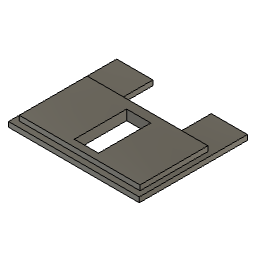
table_window (Autodesk Fusion 360 design; units mm, degrees)
Autodesk Fusion 360 part; units mm, degrees
note: some values were not read from the file. Set by a fixed rule: which sketch regions a step uses.
sketch "Sketch1" plane through (0, 0, 0) normal (0, 0, 1) x (1, 0, 0)
  line L0 (0, 0) -> (76.2, 0)
  line L1 (76.2, 0) -> (76.2, 42.8752)
  line L2 (76.2, 42.8752) -> (0, 42.8752)
  line L3 (0, 42.8752) -> (0, 0)
  line L4 (38.1, 42.8752) -> (38.1, 0) construction
  line L5 (0, 21.4376) -> (76.2, 20.5486) construction
  line L6 (30.48, 4.2545) -> (45.72, 4.2545)
  line L7 (79.375, -3.6195) -> (-3.175, -3.6195)
  line L8 (-3.175, -3.6195) -> (-3.175, 45.6057)
  line L9 (-3.175, 45.6057) -> (79.375, 45.6057)
  line L10 (79.375, 45.6057) -> (79.375, -3.6195)
  line L11 (74.796, 42.8752) -> (79.375, 45.6057) construction
  line L12 (-3.175, -3.6195) -> (2.8949, 0) construction
  line L13 (79.375, -3.6195) -> (73.3051, 0) construction
  line L14 (1.404, 42.8752) -> (-3.175, 45.6057) construction
  line L15 (45.72, 37.2745) -> (30.48, 37.2745)
  line L16 (45.72, 37.2745) -> (45.72, 4.2545)
  line L17 (30.48, 37.2745) -> (30.48, 4.2545)
  dimension "d1" = 76.2
  dimension "d2" = 42.8752
  dimension "d3" = 15.24
  dimension "d5" = 82.55
  dimension "d6" = 49.2252
  constraint horizontal L0
  constraint vertical L1
  constraint horizontal L2
  constraint vertical L3
  constraint coincident L0.start L3.end
  constraint midpoint L2 L4.start
  constraint midpoint L0 L4.end
  constraint midpoint L3 L5.start
  constraint coincident L1 L5.end
  constraint horizontal L7
  constraint perpendicular L7 L8
  constraint parallel L7 L9
  constraint parallel L8 L10
  constraint coincident L2 L11.start
  constraint collinear L11 L12
  constraint coincident L0 L12.end
  constraint coincident L0 L13.end
  constraint collinear L13 L14
  constraint coincident L2 L14.start
  constraint horizontal L15
  constraint perpendicular L6 L17
  measures "d1" distance of L0.start L0.end
  measures "d2" distance of L0.start L2.end
  measures "d3" distance of L6.start L6.end
  measures "d5" distance of L8.end L9.end
  measures "d6" distance of L7.end L8.end
extrude "Extrude1" add sketch "Sketch1" along normal blind 6.35 contours L0 L1 L2 L3
extrude "Extrude2" add sketch "Sketch1" along normal blind 3.175 contours L7 L8 L9 L10
sketch "Sketch2" plane through (0, 45.6057, 0) normal (0, 1, 0) x (-1, 0, 0)
  line L0 (-79.375, 0) -> (3.175, 0)
  line L1 (3.175, 0) -> (3.175, 3.175)
  line L2 (3.175, 3.175) -> (-79.375, 3.175)
  line L3 (-79.375, 3.175) -> (-79.375, 0)
  line L4 (3.175, 0) -> (-19.685, 0)
  line L5 (-19.685, 0) -> (-19.685, 3.175)
  line L6 (-19.685, 3.175) -> (3.175, 3.175)
  line L7 (3.175, 3.175) -> (3.175, 0)
  line L8 (-79.375, 0) -> (-56.515, 0)
  line L9 (-56.515, 0) -> (-56.515, 3.175)
  line L10 (-56.515, 3.175) -> (-79.375, 3.175)
  line L11 (-79.375, 3.175) -> (-79.375, 0)
  dimension "d12" = 22.86
  dimension "d13" = 22.86
  constraint horizontal L4
  constraint vertical L5
  constraint horizontal L6
  constraint vertical L7
  constraint coincident L0.end L1.start
  constraint horizontal L8
  constraint vertical L9
  constraint horizontal L10
  constraint vertical L11
  constraint coincident L0.start L3.end
  measures "d12" distance of L0.end L4.end
  measures "d13" distance of L0.start L8.end
extrude "Extrude3" add sketch "Sketch2" along normal blind 19.05 contours L0 L2 L3 L8 L9 L10 L11 | L0 L1 L2 L4 L5 L6 L7
